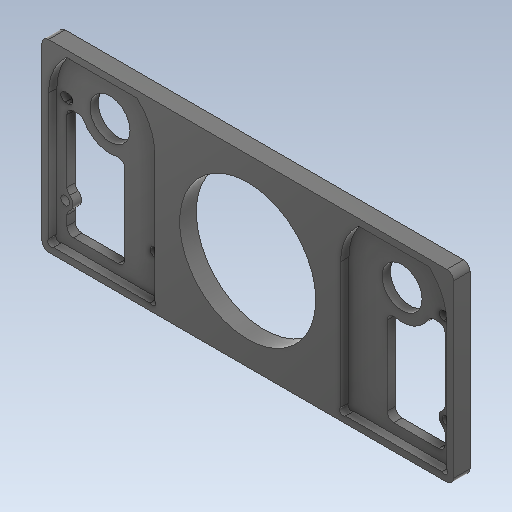
# Autodesk Inventor part: Trunk_horizontal_frame_02
Saved by Autodesk Inventor 2020.4 (Build 244396000, 396)
## iProperties
Created: 2021-09-26
Part Number: Trunk_horizontal_frame_02
Material: アセタール樹脂、黒
Document SubType Name: Modeling
Designer: Masato
Density: 1.425 g/cm^3
Appearance: 滑らか - 黒
Mass: 23.5473 g
Surface Area: 125.547 cm^2
Volume: 16.5244 cm^3
Author: Masato
Autodesk Inventor part; units mm, degrees
ref_plane "YZ Plane" through (0, 0, 0) normal (1, 0, 0) x (0, 1, 0)
ref_plane "XZ Plane" through (0, 0, 0) normal (0, 1, 0) x (-1, 0, 0)
ref_plane "XY Plane" through (0, 0, 0) normal (0, 0, 1) x (1, 0, 0)
derived "Trunk_horizontal_frame_01.ipt"
sketch "スケッチ1" plane through (0, 0, 0) normal (0, 0, 1) x (1, 0, 0)
  line L0 (-62, 30.75) -> (62, 30.75) construction
  line L1 (62, -30.75) -> (-62, -30.75) construction
  line L2 (-62, 30.75) -> (62, -30.75) construction
  line L3 (62, 30.75) -> (-62, -30.75) construction
  line L4 (0, 30.75) -> (0, -30.75) construction
  circle A0 centre (-44, 2.25) radius 10.5 construction
  line L5 (-57.5, 1.25) -> (-30.5, 1.25) construction
  line L6 (-30.5, 1.25) -> (-30.5, -25.75) construction
  line L7 (-30.5, -25.75) -> (-57.5, -25.75) construction
  line L8 (-57.5, -25.75) -> (-57.5, 1.25) construction
  line L9 (-44, 1.25) -> (-44, -25.75) construction
  line L10 (-57.5, -12.25) -> (-30.5, -12.25) construction
  circle A1 centre (-57.5, 1.25) radius 1.35 construction
  circle A2 centre (-57.5, -25.75) radius 1.35
  circle A3 centre (-30.5, 1.25) radius 1.35 construction
  circle A4 centre (-30.5, -25.75) radius 1.35
  line L11 (-27.5, 21.75) -> (-22.5, 21.75) construction
  line L12 (-22.5, 21.75) -> (-22.5, 11.75) construction
  line L13 (-22.5, 11.75) -> (-27.5, 11.75) construction
  line L14 (-27.5, 11.75) -> (-27.5, 21.75) construction
  line L15 (-27.5, 21.75) -> (-22.5, 11.75) construction
  line L16 (-22.5, 21.75) -> (-27.5, 11.75) construction
  line L17 (-27.51, 21.76) -> (-22.49, 21.76) construction
  line L18 (-22.49, 21.76) -> (-22.49, 11.74) construction
  line L19 (-22.49, 11.74) -> (-27.51, 11.74) construction
  line L20 (-27.51, 11.74) -> (-27.51, 21.76) construction
  line L21 (-27.51, 21.76) -> (-22.49, 11.74) construction
  line L22 (-22.49, 21.76) -> (-27.51, 11.74) construction
  line L23 (-27.51, 16.75) -> (-22.49, 16.75) construction
  line L24 (-25, 21.76) -> (-25, 11.74) construction
  arc A5 (-27.51, 21.76) -> (-27.51, 19.66) centre (-27.51, 20.71) ccw construction
  arc A6 (-22.49, 19.66) -> (-22.49, 21.76) centre (-22.49, 20.71) ccw construction
  arc A7 (-22.49, 11.74) -> (-22.49, 13.84) centre (-22.49, 12.79) ccw construction
  arc A8 (-27.51, 13.84) -> (-27.51, 11.74) centre (-27.51, 12.79) ccw construction
  circle A9 centre (-25, 27.75) radius 1.55 construction
  arc A10 (-27.51, -19.66) -> (-27.51, -21.76) centre (-27.51, -20.71) ccw construction
  line L25 (-22.5, -21.75) -> (-27.5, -21.75) construction
  line L26 (-22.49, -21.76) -> (-27.51, -21.76) construction
  arc A11 (-22.49, -21.76) -> (-22.49, -19.66) centre (-22.49, -20.71) ccw construction
  line L27 (-27.5, -21.75) -> (-27.5, -9.25) construction
  line L28 (-27.51, -21.76) -> (-27.51, -9.24) construction
  line L29 (-27.51, -15.5) -> (-22.49, -15.5) construction
  line L30 (-25, -9.24) -> (-25, -21.76) construction
  line L31 (-27.5, -9.25) -> (-22.5, -21.75) construction
  line L32 (-22.5, -9.25) -> (-27.5, -21.75) construction
  line L33 (-27.51, -9.24) -> (-22.49, -21.76) construction
  line L34 (-22.49, -9.24) -> (-27.51, -21.76) construction
  line L35 (-22.5, -9.25) -> (-22.5, -21.75) construction
  line L36 (-22.49, -9.24) -> (-22.49, -21.76) construction
  circle A12 centre (-25, -27.75) radius 1.55 construction
  arc A13 (-22.49, -11.34) -> (-22.49, -9.24) centre (-22.49, -10.29) ccw construction
  line L37 (-27.5, -9.25) -> (-22.5, -9.25) construction
  line L38 (-27.51, -9.24) -> (-22.49, -9.24) construction
  arc A14 (-27.51, -9.24) -> (-27.51, -11.34) centre (-27.51, -10.29) ccw construction
  circle A15 centre (-44, 2.25) radius 11 construction
  line L39 (62, 2.25) -> (-62, 2.25) construction
  line L40 (-60, 14.25) -> (-28, 14.25) construction
  line L41 (-28, 14.25) -> (-28, -28.75) construction
  line L42 (-28, -28.75) -> (-60, -28.75) construction
  line L43 (-60, -28.75) -> (-60, 14.25) construction
  line L44 (-60, 14.25) -> (-28, -28.75) construction
  line L45 (-28, 14.25) -> (-60, -28.75) construction
  line L46 (-62, 30.75) -> (-62, -30.75) construction
  line L47 (62, 30.75) -> (62, -30.75) construction
  circle A16 centre (-44, 2.25) radius 12.5 construction
  circle A17 centre (-44, 2.25) radius 20.5 construction
  circle A18 centre (-44, 2.25) radius 28.5 construction
  circle A19 centre (-44, 26.75) radius 2.2 construction
  circle A20 centre (-61.3241, 19.5741) radius 2.2 construction
  circle A21 centre (-68.5, 2.25) radius 2.2 construction
  circle A22 centre (-61.3241, -15.0741) radius 2.2 construction
  circle A23 centre (-44, -22.25) radius 2.2 construction
  circle A24 centre (-26.6759, -15.0741) radius 2.2 construction
  circle A25 centre (-19.5, 2.25) radius 2.2 construction
  circle A26 centre (-26.6759, 19.5741) radius 2.2 construction
  line L48 (-62, -21.122) -> (-62, -30.75) construction
  arc A27 (22.49, -9.24) -> (22.49, -11.34) centre (22.49, -10.29) ccw construction
  line L49 (27.51, -9.24) -> (22.49, -9.24) construction
  arc A28 (27.51, -11.34) -> (27.51, -9.24) centre (27.51, -10.29) ccw construction
  line L50 (27.51, -21.76) -> (27.51, -9.24) construction
  line L51 (22.49, -9.24) -> (22.49, -21.76) construction
  circle A29 centre (26.6759, -15.0741) radius 2.2 construction
  arc A30 (27.51, -21.76) -> (27.51, -19.66) centre (27.51, -20.71) ccw construction
  line L52 (22.49, -21.76) -> (27.51, -21.76) construction
  arc A31 (22.49, -19.66) -> (22.49, -21.76) centre (22.49, -20.71) ccw construction
  circle A32 centre (25, -27.75) radius 1.55 construction
  circle A33 centre (30.5, -25.75) radius 1.35 construction
  circle A34 centre (44, -22.25) radius 2.2 construction
  circle A35 centre (57.5, -25.75) radius 1.35
  circle A36 centre (61.3241, -15.0741) radius 2.2 construction
  line L53 (62, -21.122) -> (62, -30.75) construction
  circle A37 centre (68.5, 2.25) radius 2.2 construction
  circle A38 centre (61.3241, 19.5741) radius 2.2 construction
  circle A39 centre (44, 26.75) radius 2.2 construction
  circle A40 centre (44, 2.25) radius 11 construction
  circle A41 centre (26.6759, 19.5741) radius 2.2 construction
  circle A42 centre (25, 27.75) radius 1.55 construction
  circle A43 centre (30.5, 1.25) radius 1.35 construction
  circle A44 centre (57.5, 1.25) radius 1.35 construction
  circle A45 centre (19.5, 2.25) radius 2.2 construction
  line L54 (22.49, 11.74) -> (27.51, 11.74) construction
  arc A46 (27.51, 11.74) -> (27.51, 13.84) centre (27.51, 12.79) ccw construction
  arc A47 (22.49, 13.84) -> (22.49, 11.74) centre (22.49, 12.79) ccw construction
  line L55 (22.49, 21.76) -> (22.49, 11.74) construction
  line L56 (27.51, 11.74) -> (27.51, 21.76) construction
  arc A48 (22.49, 21.76) -> (22.49, 19.66) centre (22.49, 20.71) ccw construction
  line L57 (27.51, 21.76) -> (22.49, 21.76) construction
  arc A49 (27.51, 19.66) -> (27.51, 21.76) centre (27.51, 20.71) ccw construction
  line L58 (-68.5, 2.25) -> (-73.5, 2.25) construction
  circle A50 centre (-26.6759, -15.0741) radius 7.2 construction
  circle A51 centre (-44, 2.25) radius 24.5 construction
  circle A52 centre (-30.5, -25.75) radius 2.4 construction
  line L59 (-62, 16.25) -> (62, 16.25)
  line L60 (-60.01, 2.25) -> (-60.01, -35.7751)
  circle A53 centre (-44, 2.25) radius 6.05
  arc A54 (-54.5868, 14.26) -> (-55.1489, 13.7401) centre (-44, 2.25) ccw construction
  line L61 (-54.5868, 14.26) -> (-53.8211, 14.26) construction
  arc A55 (-53.8211, 14.26) -> (-55.1489, 13.7401) centre (-54.204, 13.2823) ccw
  arc A56 (-55.1489, 13.7401) -> (-60.01, 2.25) centre (-44, 2.25) ccw
  line L62 (-60.01, -37.26) -> (-58.5251, -37.26) construction
  arc A57 (-60.01, -35.7751) -> (-58.5251, -37.26) centre (-59.2675, -36.5175) ccw
  line L63 (-60.01, -35.7751) -> (-60.01, -37.26) construction
  line L64 (-58.5251, -37.26) -> (-29.4749, -37.26)
  arc A58 (-57.5, 2.6) -> (-57.5, -0.1) centre (-57.5, 1.25) ccw
  arc A59 (-56.5, -0.1) -> (-56.5, 2.6) centre (-56.5, 1.25) ccw
  line L65 (-57.5, 2.6) -> (-56.5, 2.6)
  line L66 (-57.5, -0.1) -> (-56.5, -0.1)
  line L67 (-27.99, 2.25) -> (-27.99, -35.7751)
  arc A60 (-32.8511, 13.7401) -> (-34.1789, 14.26) centre (-33.796, 13.2823) ccw
  arc A61 (-27.99, 2.25) -> (-32.8511, 13.7401) centre (-44, 2.25) ccw
  arc A62 (-29.4749, -37.26) -> (-27.99, -35.7751) centre (-28.7325, -36.5175) ccw
  line L68 (-53.8211, 14.26) -> (-34.1789, 14.26)
  arc A63 (-52.3331, -1.15) -> (-39.5, -5.5442) centre (-44, 2.25) ccw
  line L69 (-52.3331, -1.15) -> (-57, -1.15)
  line L70 (-57, -1.15) -> (-57, -23.4027)
  line L71 (60.01, 2.25) -> (60.01, -35.7751)
  circle A64 centre (44, 2.25) radius 6.05
  arc A65 (55.1489, 13.7401) -> (53.8211, 14.26) centre (54.204, 13.2823) ccw
  arc A66 (60.01, 2.25) -> (55.1489, 13.7401) centre (44, 2.25) ccw
  arc A67 (58.5251, -37.26) -> (60.01, -35.7751) centre (59.2675, -36.5175) ccw
  line L72 (58.5251, -37.26) -> (29.4749, -37.26)
  arc A68 (57.5, -0.1) -> (57.5, 2.6) centre (57.5, 1.25) ccw
  arc A69 (56.5, 2.6) -> (56.5, -0.1) centre (56.5, 1.25) ccw
  line L73 (57.5, 2.6) -> (56.5, 2.6)
  arc A70 (32.8511, 13.7401) -> (27.99, 2.25) centre (44, 2.25) ccw
  arc A71 (34.1789, 14.26) -> (32.8511, 13.7401) centre (33.796, 13.2823) ccw
  line L74 (27.99, 2.25) -> (27.99, -35.7751)
  arc A72 (27.99, -35.7751) -> (29.4749, -37.26) centre (28.7325, -36.5175) ccw
  line L75 (53.8211, 14.26) -> (34.1789, 14.26)
  arc A73 (39.5, -5.5442) -> (52.3331, -1.15) centre (44, 2.25) ccw
  line L76 (52.3331, -1.15) -> (57, -1.15)
  line L77 (57, -1.15) -> (57, -23.4027)
  line L78 (57.5, -0.1) -> (56.5, -0.1)
  circle A74 centre (0, -11.5) radius 20.5
  arc A75 (-57, -28.0973) -> (-57, -23.4027) centre (-57.5, -25.75) ccw
  line L79 (-57, -28.0973) -> (-57, -34.25)
  line L80 (-57, -34.25) -> (-39.5, -34.25)
  line L81 (-39.5, -34.25) -> (-39.5, -5.5442)
  arc A76 (57, -23.4027) -> (57, -28.0973) centre (57.5, -25.75) ccw
  line L82 (57, -28.0973) -> (57, -34.25)
  line L83 (57, -34.25) -> (39.5, -34.25)
  line L84 (39.5, -34.25) -> (39.5, -5.5442)
  line L85 (-62, 16.25) -> (-62, -39.25)
  line L86 (-62, -39.25) -> (62, -39.25)
  line L87 (62, -39.25) -> (62, 16.25)
  line L88 (-60, -37.25) -> (-28, -37.25) construction
  arc A77 (-48.9902, 27.0632) -> (-58.017, 23.3242) centre (-44, 2.25) ccw
  arc A78 (-41, 30.75) -> (-48.9902, 27.0632) centre (-44, 26.75) ccw
  arc A79 (-58.017, 23.3242) -> (-65.0742, 16.267) centre (-61.3241, 19.5741) ccw
  arc A80 (-65.0742, 16.267) -> (-68.8132, 7.2402) centre (-44, 2.25) ccw
  arc A81 (-68.8132, 7.2402) -> (-68.8132, -2.7402) centre (-68.5, 2.25) ccw
  arc A82 (-68.8132, -2.7402) -> (-65.0742, -11.767) centre (-44, 2.25) ccw
  arc A83 (-65.0742, -11.767) -> (-62, -20.0282) centre (-61.3241, -15.0741) ccw
  line L89 (-62, -20.0282) -> (-62, -21.122)
  arc A84 (48.9902, 27.0632) -> (41, 30.75) centre (44, 26.75) ccw
  arc A85 (58.017, 23.3242) -> (48.9902, 27.0632) centre (44, 2.25) ccw
  arc A86 (65.0742, 16.267) -> (58.017, 23.3242) centre (61.3241, 19.5741) ccw
  arc A87 (68.8132, 7.2402) -> (65.0742, 16.267) centre (44, 2.25) ccw
  arc A88 (68.8132, -2.7402) -> (68.8132, 7.2402) centre (68.5, 2.25) ccw
  arc A89 (65.0742, -11.767) -> (68.8132, -2.7402) centre (44, 2.25) ccw
  arc A90 (62, -20.0282) -> (65.0742, -11.767) centre (61.3241, -15.0741) ccw
  line L90 (62, -20.0282) -> (62, -21.122)
  line L91 (19.5, 27.75) -> (-19.5, 27.75)
  line L92 (-19.5, 27.75) -> (-19.5, 7.25)
  circle A91 centre (-25, 27.75) radius 2.75 construction
  line L93 (-14.7303, 3.75) -> (14.7303, 3.75)
  arc A92 (-14.7303, 3.75) -> (-19.5, 7.25) centre (-19.5, 2.25) ccw
  line L94 (19.5, 27.75) -> (19.5, 7.25)
  arc A93 (19.5, 7.25) -> (14.7303, 3.75) centre (19.5, 2.25) ccw
  arc A94 (-19.5, -2.75) -> (-14.7303, 0.75) centre (-19.5, 2.25) ccw
  line L95 (-14.7303, 0.75) -> (14.7303, 0.75)
  arc A95 (14.7303, 0.75) -> (19.5, -2.75) centre (19.5, 2.25) ccw
  line L96 (-19.5, -2.75) -> (-19.5, -27.75)
  line L97 (-19.5, -27.75) -> (19.5, -27.75)
  line L98 (19.5, -27.75) -> (19.5, -2.75)
  point P0 (0, 0)
  point P1 (-25, 16.75)
  point P2 (-25, -15.5)
  point P3 (-44, -7.25)
  point P4 (28, -28.75)
  dimension "d6" = 12.1
  dimension "d7" = 0.01
  dimension "d9" = 0.01
  dimension "d10" = 1.05
  dimension "d11" = 1.05
  dimension "d13" = 1
  dimension "d14" = 16.01
  dimension "d16" = 9
  dimension "d17" = 2.4
  dimension "d18" = 5
  dimension "d21" = 2
  dimension "d22" = 2
  dimension "d24" = 7.25
  dimension "d26" = 41
  dimension "d27" = 2.4
  dimension "d29" = 8.5
  dimension "d30" = 0.01
  dimension "d31" = 2
  dimension "d32" = 5
  dimension "d33" = 12
  dimension "d34" = 2
  dimension "d35" = 55.5
  measures "d6" diameter of A53
  measures "d7" distance between parallel lines of L60 L43
  measures "d9" distance between parallel lines of L40 L61
  measures "d10" radius of A55
  measures "d11" radius of A57
  measures "d13" distance of A1.centre A59.centre
  measures "d14" radius of A56
  measures "d16" radius of A63
  measures "d17" vertical distance of L69.end A59.centre
  measures "d18" horizontal distance of L1.end L70.end
  measures "d21" horizontal distance of L59.start L40.start
  measures "d22" horizontal distance of L59.start L40.start
  measures "d24" distance edge to line of A74 L59
  measures "d26" diameter of A74
  measures "d27" radius of A75
  measures "d29" distance of L88.start L42.end
  measures "d30" horizontal distance of L62.start L88.start
  measures "d31" horizontal distance of L85.end L88.start
  measures "d32" horizontal distance of L85.end L79.end
  measures "d33" distance between parallel lines of L27 L81
  measures "d34" distance edge to line of A74 L35
  measures "d35" distance of L85.end L59.start
extrude "押し出し1" add sketch "スケッチ1" along normal blind 5 contours L59 L92 A92 L93 A74 A94 L96 L97 L98 A95 A93 L94 L87 L86 L85 | L59 L94 A93 L93 A74 A92 L92 | A74 L96 A94 | A95 L98 A74 | A74 L97 L96 | L98 L97 A74
extrude "押し出し2" add sketch "スケッチ1" along normal blind 2.5 contours A56 A55 L68 A60 A61 L67 A62 L64 A57 L60 | L71 A67 L72 A72 L74 A70 A71 L75 A65 A66
fillet "フィレット1" radius 2 18 edges at (-62, 16.25, 2.5) (-62, -39.25, 2.5) (-52.3331, -1.15, 1.25) (-57, -1.15, 1.25) (-39.5, -5.5442, 1.25) (-39.5, -34.25, 1.25) (-57, -34.25, 1.25) (39.5, -34.25, 1.25) (39.5, -5.5442, 1.25) (62, -39.25, 2.5) (62, 16.25, 2.5) (52.3331, -1.15, 1.25) (57, -1.15, 1.25) (57, -34.25, 1.25) (-57, -23.4027, 1.25) (-57, -28.0973, 1.25) (57, -23.4027, 1.25) (57, -28.0973, 1.25)
equation "\"d9\" = d7"
equation "\"d21\" = d22"
equation "\"d24\" = -0.5 * d26 + 0.5 * d35"
equation "\"d30\" = d7"
equation "\"d31\" = d22"
equation "\"d32\" = d18"
equation "\"d34\" = d22"
